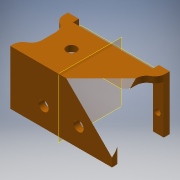
# Autodesk Inventor part: Servo_vice
Saved by Autodesk Inventor 2016 (Build 200138000, 138)
## iProperties
Created: 2015-10-07
Part Number: Servo_vice
Material: Generic
Document SubType Name: Modeling
Designer: powasar16
Density: 1 g/cm^3
Appearance: Default
Author: powasar16
Autodesk Inventor part; units mm, degrees
ref_plane "YZ Plane" through (0, 0, 0) normal (1, 0, 0) x (0, 1, 0)
ref_plane "XZ Plane" through (0, 0, 0) normal (0, 1, 0) x (-1, 0, 0)
ref_plane "XY Plane" through (0, 0, 0) normal (0, 0, 1) x (1, 0, 0)
sketch "Sketch1" plane through (0, 0, 0) normal (0, 0, 1) x (1, 0, 0)
  line L0 (-4.3, 0) -> (27.3, 0) projected
  line L1 (27.5, -0.2) -> (27.5, -5.5) projected
  line L2 (-4.3, -12) -> (27.3, -12) projected
  line L3 (27.5, -6.5) -> (27.5, -11.8) projected
  line L4 (-4.5, -0.2) -> (-4.5, -5.5) projected
  line L5 (-4.5, -6.5) -> (-4.5, -11.8) projected
  line L6 (-4.5, 0) -> (-1.071, 0)
  line L7 (-1.071, 0) -> (-1.071, -12)
  line L8 (-1.071, -12) -> (-4.5, -12)
  line L9 (-4.5, -12) -> (-4.5, 0)
  arc A0 (-3.366, -6.5) -> (-3.366, -5.5) centre (-2.5, -6) ccw projected
  circle A1 centre (-2.5, -6) radius 1
  line L10 (27.5, -12) -> (24.071, -12)
  line L11 (24.071, -12) -> (24.071, 0)
  line L12 (24.071, 0) -> (27.5, 0)
  line L13 (27.5, 0) -> (27.5, -12)
  arc A2 (26.366, -5.5) -> (26.366, -6.5) centre (25.5, -6) ccw projected
  circle A3 centre (25.5, -6) radius 1
  line L14 (-1.071, 0) -> (-4.5, 0)
  line L15 (-4.5, 0) -> (-4.5, 1.905)
  line L16 (-4.5, 1.905) -> (-1.071, 1.905)
  line L17 (-1.071, 1.905) -> (-1.071, 0)
  line L18 (11.5, 0) -> (11.5, -12) construction
  line L19 (27.5, 0) -> (24.071, 0)
  line L20 (24.071, 0) -> (27.5, 0)
  line L21 (27.5, 0) -> (27.5, 1.905)
  line L22 (27.5, 1.905) -> (24.071, 1.905)
  line L23 (24.071, 1.905) -> (24.071, 0)
  line L24 (-4.5, 1.905) -> (-1.071, 1.905)
  line L25 (-1.071, 1.905) -> (-1.071, 5.08)
  line L26 (-1.071, 5.08) -> (-4.5, 5.08)
  line L27 (-4.5, 5.08) -> (-4.5, 1.905)
  line L28 (24.071, 1.905) -> (27.5, 1.905)
  line L29 (27.5, 1.905) -> (27.5, 5.08)
  line L30 (27.5, 5.08) -> (24.071, 5.08)
  line L31 (24.071, 5.08) -> (24.071, 1.905)
  point P0 (0, 0)
  dimension "d0" = 3.429
  dimension "d1" = 3.429
  dimension "d2" = 1.905
  dimension "d8" = 3.175
  dimension "d9" = 3.175
  constraints: 52 end point, 10 parallel, 5 collinear, 5 horizontal, 5 perpendicular, 4 point on line, 4 symmetric about line, 2 coincident, 2 midpoint, 1 centre point, 1 concentric, 3 other
  measures "d0" distance between parallel lines of L7 L4
  measures "d1" distance between parallel lines of L1 L11
  measures "d2" distance between parallel lines of L0 L16
  measures "d8" distance between parallel lines of L24 L26
  measures "d9" distance of L28.end L29.end
extrude "Extrusion1" add sketch "Sketch1" along normal blind 1.905 contours L6 L15 L16 L17 L0 | L0 L7 L2 L8 L9 L5 L4 L6 | L23 L22 L21 L12 L0 | L0 L12 L13 L1 L3 L10 L2 L11 | L16 L27 L26 L25 | L31 L30 L29 L22
ref_plane "Work Plane1" through (0, 3.175, 15) normal (0, 1, 0) x (1, 0, 0)
sketch "Sketch2" plane through (0, 3.175, 15) normal (0, 1, 0) x (1, 0, 0)
  line L0 (-1.071, 15) -> (-4.5, 15) projected
  line L1 (-4.5, 15) -> (-4.5, 13.095) projected
  line L2 (-1.071, 13.095) -> (-4.5, 13.095) projected
  line L3 (-1.071, 15) -> (-1.071, 13.095) projected
  line L4 (27.5, 15) -> (24.071, 15) projected
  line L5 (24.071, 15) -> (24.071, 13.095) projected
  line L6 (27.5, 13.095) -> (24.071, 13.095) projected
  line L7 (27.5, 15) -> (27.5, 13.095) projected
  line L8 (22.8, 0) -> (0.2, 0) projected
  line L9 (-4.5, 13.095) -> (27.5, 13.095)
  line L10 (27.5, -3.175) -> (-4.5, -3.175)
  line L11 (-4.5, 11.19) -> (-1.071, 11.19)
  line L12 (-1.071, 11.19) -> (-1.071, 0)
  line L13 (-1.071, 0) -> (-4.5, 0)
  line L14 (27.5, 0) -> (24.071, 0)
  line L15 (24.071, 0) -> (24.071, 11.19)
  line L16 (24.071, 11.19) -> (27.5, 11.19)
  line L17 (23, 15) -> (23, 5) projected
  line L18 (0, 5) -> (0, 15) projected
  line L19 (-1.071, 15) -> (-1.071, 13.095) projected
  line L20 (24.071, 15) -> (24.071, 13.095) projected
  arc A0 (-1.071, 7.761) -> (-4.5, 11.19) centre (-4.5, 7.761) ccw
  arc A1 (-4.5, 0) -> (-1.071, 3.429) centre (-4.5, 3.429) ccw
  arc A2 (27.5, 11.19) -> (24.071, 7.761) centre (27.5, 7.761) ccw
  arc A3 (24.071, 3.429) -> (27.5, 0) centre (27.5, 3.429) ccw
  line L21 (-4.5, -3.175) -> (-4.5, 0)
  line L22 (-4.5, 11.19) -> (-4.5, 13.095)
  line L23 (27.5, 13.095) -> (27.5, 11.19)
  line L24 (27.5, 0) -> (27.5, -3.175)
  dimension "d5" = 3.175
  dimension "d13" = 1.905
  constraints: 24 end point, 8 point on circle, 8 tangent, 7 parallel, 6 collinear, 6 point on line, 4 centre point, 4 perpendicular, 3 horizontal
  measures "d5" distance between parallel lines of L8 L10
  measures "d13" distance between parallel lines of L2 L11
extrude "Extrusion2" add sketch "Sketch2" along normal blind 1.905 contours L9 L6 L23 L16 L15 L14 L24 L10 L21 L13 L12 L11 L22 L2 | L11 L12 A0 | L12 L13 A1 | A2 L15 L16 | A3 L14 L15
sketch "Sketch6" plane through (0, 3.175, 15) normal (0, -1, 0) x (1, 0, 0)
  line L0 (0.2, 0) -> (22.8, 0) projected
  line L1 (-4.5, -15) -> (-4.5, 3.175) projected
  line L2 (27.5, 3.175) -> (-4.5, 3.175)
  line L3 (-4.5, 3.175) -> (-4.5, 1.27)
  line L4 (-4.5, 1.27) -> (27.5, 1.27)
  line L5 (27.5, 1.27) -> (27.5, 3.175)
  line L6 (27.5, 3.175) -> (27.5, -13.095) projected
  line L7 (-4.5, 3.175) -> (27.5, 3.175) projected
  point P0 (0, -15)
  dimension "d10" = 1.905
  constraints: 8 end point, 2 collinear, 2 parallel, 1 horizontal, 1 perpendicular, 1 point on line
  measures "d10" distance between parallel lines of L2 L4
extrude "Extrusion3" add sketch "Sketch6" along normal up to surface (15.175 mm away)
fillet "Fillet1" radius 3.175 4 edges at (-4.5, 4.1275, 3.81) (-4.5, 4.1275, 15) (27.5, 4.1275, 15) (27.5, 4.1275, 3.81)
sketch "Sketch7" plane through (-4.5, 5.08, 18.175) normal (0, 0, 1) x (1, 0, 0)
  line L0 (32, -17.08) -> (32, 0) projected
  line L1 (0, 0) -> (32, 0) projected
  line L2 (0, -17.08) -> (0, 0) projected
  line L3 (0, -17.08) -> (32, -17.08) projected
  line L4 (31.8064, -17.08) -> (0.1936, -17.08) construction
  line L5 (32, -17.08) -> (32, 0) construction
  circle A0 centre (10.5, -11.08) radius 1.5875
  circle A1 centre (10.5, -11.08) radius 3.75
  point P0 (4.5, -5.08)
  dimension "d15" = 3.175
  constraints: 2 centre point, 1 concentric, 2 other
  measures "d15" diameter of A0
sketch "Sketch8" plane through (24.071, 5.08, 0) normal (0, 1, 0) x (1, 0, 0)
  arc A0 (1.7804, -4.2323) -> (3.429, -1.4483) centre (0.254, -1.4483) ccw projected
  line L0 (3.429, 0) -> (3.429, -1.4483) projected
  line L1 (3.429, 0) -> (0, 0) projected
  line L2 (0, 0) -> (0, -1.905) projected
  line L3 (0, -1.905) -> (-25.142, -1.905) projected
  line L4 (-25.142, 0) -> (-25.142, -1.905) projected
  line L5 (-25.142, 0) -> (-28.571, 0) projected
  line L6 (-28.571, 0) -> (-28.571, -1.4483) projected
  arc A1 (-28.571, -1.4483) -> (-26.9224, -4.2323) centre (-25.396, -1.4483) ccw projected
  arc A2 (-25.142, -7.239) -> (-26.9224, -4.2323) centre (-28.571, -7.239) ccw projected
  line L7 (-25.142, -7.239) -> (-25.142, -11.571) projected
  arc A3 (-26.9224, -14.5777) -> (-25.142, -11.571) centre (-28.571, -11.571) ccw projected
  arc A4 (-26.9224, -14.5777) -> (-28.571, -17.3617) centre (-25.396, -17.3617) ccw projected
  line L8 (-28.571, -17.3617) -> (-28.571, -18.175) projected
  line L9 (-28.571, -18.175) -> (3.429, -18.175) projected
  line L10 (3.429, -18.175) -> (3.429, -17.3617) projected
  arc A5 (3.429, -17.3617) -> (1.7804, -14.5777) centre (0.254, -17.3617) ccw projected
  arc A6 (0, -11.571) -> (1.7804, -14.5777) centre (3.429, -11.571) ccw projected
  line L11 (0, -11.571) -> (0, -7.239) projected
  arc A7 (1.7804, -4.2323) -> (0, -7.239) centre (3.429, -7.239) ccw projected
  line L12 (-25.142, -7.239) -> (-25.142, -11.571) construction
  circle A8 centre (-18.071, -9.405) radius 1.5875
  line L13 (-21.821, 16.1332) -> (-14.321, 16.1332)
  line L14 (-18.071, 16.1332) -> (-18.071, -9.3987) construction
  line L15 (-25.142, -9.405) -> (0, -9.405) construction
  point P0 (-24.071, 0)
  dimension "d16" = 3.175
  constraints: 6 end point, 3 midpoint, 2 point on line, 1 centre point, 1 horizontal, 1 vertical, 2 other
  measures "d16" diameter of A8
extrude "Extrusion4" cut sketch "Sketch8" against normal up to next contours A8
extrude "Extrusion5" cut sketch "Sketch7" against normal up to next contours A0
ref_plane "Work Plane3" through (11.5, -12, 0) normal (1, 0, 0) x (0, 0, -1)
mirror "Mirror1" about plane through (11.5, -12, 0) normal (1, 0, 0) of "Extrusion5"
body "Solid1"
